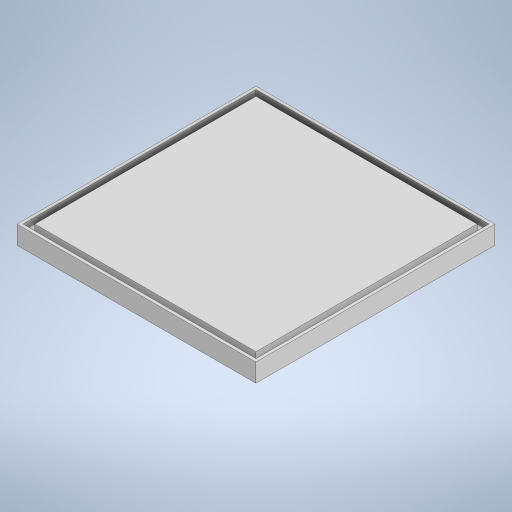
# Autodesk Inventor part: 사각형 OV-PAM 5패턴 상단
Saved by Autodesk Inventor 2024 (Build 280153000, 153)
## iProperties
Created: 2023-06-16
Part Number: 사각형 OV-PAM 5패턴 상단
Material: 일반
Document SubType Name: Modeling
Designer: jsw
Density: 1 g/cm^3
Appearance: 기본값
Author: jsw
Autodesk Inventor part; units mm, degrees
ref_plane "YZ Plane" through (0, 0, 0) normal (1, 0, 0) x (0, 1, 0)
ref_plane "XZ Plane" through (0, 0, 0) normal (0, 1, 0) x (-1, 0, 0)
ref_plane "XY Plane" through (0, 0, 0) normal (0, 0, 1) x (1, 0, 0)
sketch "스케치1" plane through (0, 0, 0) normal (0, 1, 0) x (-1, 0, 0)
  line L0 (0, 0) -> (64.8, 0)
  line L1 (64.8, 0) -> (64.8, -64.8)
  line L2 (64.8, -64.8) -> (0, -64.8)
  line L3 (0, -64.8) -> (0, 0)
  dimension "d0" = 64.8
  dimension "d1" = 64.8
  constraints: 8 end point, 2 parallel, 1 horizontal, 1 perpendicular
  measures "d0" distance of L2.end L0.start
  measures "d1" distance of L0.start L0.end
extrude "돌출1" add sketch "스케치1" along normal blind 5
sketch "스케치2" plane through (0, 5, 0) normal (0, 1, 0) x (1, 0, 0)
  line L0 (-2.4, 2.4) -> (-62.4, 2.4)
  line L1 (-62.4, 2.4) -> (-62.4, 62.4)
  line L2 (-62.4, 62.4) -> (-2.4, 62.4)
  line L3 (-2.4, 62.4) -> (-2.4, 2.4)
  line L4 (-64.8, 0) -> (0, 0) projected
  line L5 (0, 0) -> (0, 64.8) projected
  line L6 (-64, 0.8) -> (-0.8, 0.8)
  line L7 (-0.8, 0.8) -> (-0.8, 64)
  line L8 (-0.8, 64) -> (-64, 64)
  line L9 (-64, 64) -> (-64, 0.8)
  line L10 (0, 64.8) -> (-64.8, 64.8) projected
  dimension "d54" = 60
  dimension "d55" = 1.6
  dimension "d56" = 1.6
  dimension "d57" = 1.6
  dimension "d58" = 1.6
  dimension "d59" = 2.4
  dimension "d60" = 2.4
  dimension "d61" = 2.4
  constraints: 16 end point, 4 parallel, 2 horizontal, 2 perpendicular
  measures "d54" distance of L1.end L2.end
  measures "d55" distance between parallel lines of L7 L3
  measures "d56" distance between parallel lines of L1 L9
  measures "d57" distance between parallel lines of L2 L8
  measures "d58" distance between parallel lines of L6 L0
  measures "d59" distance between parallel lines of L10 L2
  measures "d60" distance between parallel lines of L4 L0
  measures "d61" distance between parallel lines of L3 L5
extrude "돌출2" cut sketch "스케치2" against normal blind 1.6
sketch "스케치7" plane through (0, 0, 0) normal (0, -1, 0) x (1, 0, 0)
  line L0 (-29.9, -22.4) -> (-24.9, -22.4)
  line L1 (-24.9, -22.4) -> (-24.9, -42.4)
  line L2 (-24.9, -42.4) -> (-29.9, -42.4)
  line L3 (-29.9, -42.4) -> (-29.9, -22.4)
  line L4 (-39.9, -22.4) -> (-34.9, -22.4)
  line L5 (-34.9, -22.4) -> (-34.9, -42.4)
  line L6 (-34.9, -42.4) -> (-39.9, -42.4)
  line L7 (-39.9, -42.4) -> (-39.9, -22.4)
  line L8 (0, 0) -> (0, -64.8) projected
  line L9 (-34.9, -42.4) -> (-29.9, -42.4)
  line L10 (-64.8, 0) -> (0, 0) projected
  point P0 (0, -32.4)
  point P1 (-24.9, -32.4)
  point P2 (-32.4, -42.4)
  point P3 (-32.4, 0)
  dimension "d37" = 5
  dimension "d38" = 20
  dimension "d41" = 10
  constraints: 18 end point, 4 midpoint, 3 horizontal, 2 parallel, 1 collinear, 1 horizontal alignment, 1 perpendicular, 1 vertical alignment, 7 other
  measures "d37" distance of L1.end L2.end
  measures "d38" distance of L0.end L1.end
  measures "d41" distance of L0.start L4.start
extrude "돌출7" add sketch "스케치7" along normal blind 10
sketch "스케치8" plane through (-24.9, 0, -22.4) normal (1, 0, 0) x (0, 0, -1)
  circle A0 centre (6.0516, -5) radius 1.25
  circle A1 centre (13.9484, -5) radius 1.25
  line L0 (13.9484, -5) -> (6.0516, -5)
  line L1 (-22.4, 0) -> (42.4, 0) projected
  line L2 (0, 0) -> (0, -10) projected
  point P0 (10, -5)
  point P1 (10, 0)
  point P2 (0, -5)
  dimension "d48" = 2.5
  dimension "d49" = 2.5
  constraints: 3 midpoint, 2 centre point, 2 end point, 2 horizontal alignment, 1 horizontal, 1 vertical alignment
  measures "d48" diameter of A0
  measures "d49" diameter of A1
extrude "돌출8" cut sketch "스케치8" against normal blind 15
